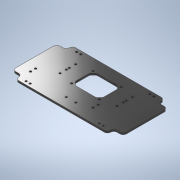
# Autodesk Inventor part: Sole_frame
Saved by Autodesk Inventor 2022.3 (Build 263350000, 350)
## iProperties
Part Number: Sole_frame
Material: GFRP
Document SubType Name: Modeling
Designer: Masato Kubotera
Density: 1.75 g/cm^3
Appearance: 低 光沢 - 黒
Description: GFRP T3
Mass: 67.4649 g
Surface Area: 284.007 cm^2
Volume: 38.5514 cm^3
Author: Masato Kubotera
Revision Number: Rev.2 Specifications for RoboCup 2023: The shape was changed for the installation of load cells.
Autodesk Inventor part; units mm, degrees
ref_plane "YZ Plane" through (0, 0, 0) normal (1, 0, 0) x (0, 1, 0)
ref_plane "XZ Plane" through (0, 0, 0) normal (0, 1, 0) x (-1, 0, 0)
ref_plane "XY Plane" through (0, 0, 0) normal (0, 0, 1) x (1, 0, 0)
sketch "スケッチ1" plane through (0, 0, 0) normal (0, 0, 1) x (1, 0, 0)
  line L0 (-96.735, 64.25) -> (78.265, 64.25)
  line L1 (78.265, 64.25) -> (78.265, -25.75)
  line L2 (78.265, -25.75) -> (-96.735, -25.75)
  line L3 (-96.735, -25.75) -> (-96.735, 64.25)
  line L4 (-96.735, 64.25) -> (78.265, -25.75) construction
  line L5 (78.265, 64.25) -> (-96.735, -25.75) construction
  line L6 (-96.735, 19.25) -> (78.265, 19.25) construction
  line L7 (-96.735, 0) -> (78.265, 0) construction
  line L8 (-80, 4) -> (-80, -4) construction
  circle A0 centre (-80, -4) radius 1.6
  line L9 (0, 64.25) -> (0, -25.75) construction
  line L10 (19, -4) -> (19, 4) construction
  circle A1 centre (19, -4) radius 1.6
  circle A2 centre (-80, 4) radius 1.6
  circle A3 centre (19, 4) radius 1.6
  line L11 (16, 12.5) -> (22, 12.5) construction
  line L12 (22, 12.5) -> (22, -12.5) construction
  line L13 (22, -12.5) -> (16, -12.5) construction
  line L14 (16, -12.5) -> (16, 12.5) construction
  line L15 (16, 12.5) -> (22, -12.5) construction
  line L16 (22, 12.5) -> (16, -12.5) construction
  line L17 (-83, 12.5) -> (-77, 12.5) construction
  line L18 (-77, 12.5) -> (-77, -12.5) construction
  line L19 (-77, -12.5) -> (-83, -12.5) construction
  line L20 (-83, -12.5) -> (-83, 12.5) construction
  line L21 (-83, 12.5) -> (-77, -12.5) construction
  line L22 (-77, 12.5) -> (-83, -12.5) construction
  line L23 (-67, 49.25) -> (6, 49.25) construction
  line L24 (6, 49.25) -> (6, -10.75) construction
  line L25 (6, -10.75) -> (-67, -10.75) construction
  line L26 (-67, -10.75) -> (-67, 49.25) construction
  line L27 (-67, 49.25) -> (6, -10.75) construction
  line L28 (6, 49.25) -> (-67, -10.75) construction
  line L29 (-83, -4.5) -> (-83, 20.5) construction
  line L30 (-83, 20.5) -> (-77, 20.5) construction
  line L31 (-77, 20.5) -> (-77, -4.5) construction
  line L32 (-77, -4.5) -> (-83, -4.5) construction
  circle A4 centre (-80, 12) radius 1.6
  circle A5 centre (-80, 4) radius 1.6
  line L33 (16, 20.5) -> (22, 20.5) construction
  line L34 (16, -4.5) -> (16, 20.5) construction
  line L35 (22, -4.5) -> (16, -4.5) construction
  line L36 (22, 20.5) -> (22, -4.5) construction
  circle A6 centre (19, 4) radius 1.6
  circle A7 centre (19, 12) radius 1.6
  line L37 (-83, 3.5) -> (-83, 28.5) construction
  line L38 (-83, 28.5) -> (-77, 28.5) construction
  line L39 (-77, 28.5) -> (-77, 3.5) construction
  line L40 (-77, 3.5) -> (-83, 3.5) construction
  circle A8 centre (-80, 20) radius 1.6
  circle A9 centre (-80, 12) radius 1.6
  line L41 (16, 28.5) -> (22, 28.5) construction
  line L42 (16, 3.5) -> (16, 28.5) construction
  line L43 (22, 3.5) -> (16, 3.5) construction
  line L44 (22, 28.5) -> (22, 3.5) construction
  circle A10 centre (19, 12) radius 1.6
  circle A11 centre (19, 20) radius 1.6
  circle A12 centre (-80, -12) radius 1.6
  line L45 (-77, -20.5) -> (-83, -20.5) construction
  line L46 (-83, -20.5) -> (-83, 4.5) construction
  line L47 (-77, 4.5) -> (-77, -20.5) construction
  line L48 (16, -20.5) -> (16, 4.5) construction
  circle A13 centre (19, -12) radius 1.6
  line L49 (22, -20.5) -> (16, -20.5) construction
  line L50 (22, 4.5) -> (22, -20.5) construction
  line L51 (45.415, -24.7) -> (77.215, -24.7) construction
  line L52 (77.215, -16.8) -> (45.415, -16.8) construction
  line L53 (45.415, -16.8) -> (45.415, -24.7) construction
  line L54 (45.415, -24.7) -> (77.215, -16.8) construction
  line L55 (77.215, -24.7) -> (45.415, -16.8) construction
  line L56 (77.215, -20.75) -> (45.415, -20.75) construction
  line L57 (61.315, -24.7) -> (61.315, -16.8) construction
  circle A14 centre (45.415, -20.75) radius 1.6
  circle A15 centre (51.765, -20.75) radius 1.6
  line L58 (73.615, -19.1623) -> (73.615, -22.3377) construction
  line L59 (73.615, -22.3377) -> (70.865, -23.9254) construction
  line L60 (70.865, -23.9254) -> (68.115, -22.3377) construction
  line L61 (68.115, -22.3377) -> (68.115, -19.1623) construction
  line L62 (68.115, -19.1623) -> (70.865, -17.5746) construction
  line L63 (70.865, -17.5746) -> (73.615, -19.1623) construction
  line L64 (-9.235, 64.25) -> (-9.235, -25.75) construction
  circle A16 centre (45.415, 59.25) radius 1.6
  circle A17 centre (51.765, 59.25) radius 1.6
  line L65 (73.615, 57.6623) -> (73.615, 60.8377) construction
  line L66 (73.615, 60.8377) -> (70.865, 62.4254) construction
  line L67 (70.865, 62.4254) -> (68.115, 60.8377) construction
  line L68 (68.115, 60.8377) -> (68.115, 57.6623) construction
  line L69 (68.115, 57.6623) -> (70.865, 56.0746) construction
  line L70 (70.865, 56.0746) -> (73.615, 57.6623) construction
  circle A18 centre (-63.885, -20.75) radius 1.6
  circle A19 centre (-70.235, -20.75) radius 1.6
  line L71 (-92.085, -19.1623) -> (-92.085, -22.3377) construction
  line L72 (-92.085, -22.3377) -> (-89.335, -23.9254) construction
  line L73 (-89.335, -23.9254) -> (-86.585, -22.3377) construction
  line L74 (-86.585, -22.3377) -> (-86.585, -19.1623) construction
  line L75 (-86.585, -19.1623) -> (-89.335, -17.5746) construction
  line L76 (-89.335, -17.5746) -> (-92.085, -19.1623) construction
  circle A20 centre (-63.885, 59.25) radius 1.6
  circle A21 centre (-70.235, 59.25) radius 1.6
  line L77 (-86.585, 57.6623) -> (-89.335, 56.0746) construction
  line L78 (-86.585, 60.8377) -> (-86.585, 57.6623) construction
  line L79 (-89.335, 62.4254) -> (-86.585, 60.8377) construction
  line L80 (-92.085, 60.8377) -> (-89.335, 62.4254) construction
  line L81 (-92.085, 57.6623) -> (-92.085, 60.8377) construction
  line L82 (-89.335, 56.0746) -> (-92.085, 57.6623) construction
  line L83 (-34.235, 49.25) -> (15.765, 49.25) construction
  line L84 (15.765, 49.25) -> (15.765, 9.25) construction
  line L85 (15.765, 9.25) -> (-34.235, 9.25) construction
  line L86 (-34.235, 9.25) -> (-34.235, 49.25) construction
  line L87 (-34.235, 49.25) -> (15.765, 9.25) construction
  line L88 (15.765, 49.25) -> (-34.235, 9.25) construction
  line L89 (-31.235, 46.25) -> (12.765, 46.25) construction
  line L90 (12.765, 46.25) -> (12.765, 12.25) construction
  line L91 (12.765, 12.25) -> (-31.235, 12.25) construction
  line L92 (-31.235, 12.25) -> (-31.235, 46.25) construction
  line L93 (-31.235, 46.25) -> (12.765, 12.25) construction
  line L94 (12.765, 46.25) -> (-31.235, 12.25) construction
  circle A22 centre (-31.235, 12.25) radius 1.6
  circle A23 centre (-31.235, 46.25) radius 1.6
  circle A24 centre (12.765, 46.25) radius 1.6
  circle A25 centre (12.765, 12.25) radius 1.6
  line L95 (-62, -21.85) -> (-61.735, -21.85)
  line L96 (77.215, -16.8) -> (77.215, -24.7) construction
  line L97 (63.465, -25.75) -> (63.465, -15.75)
  line L98 (63.465, -15.75) -> (78.265, -15.75)
  line L99 (70.865, -23.9254) -> (70.865, -17.5746) construction
  line L100 (63.465, 64.25) -> (63.465, 54.25)
  line L101 (63.465, 54.25) -> (78.265, 54.25)
  line L102 (-81.935, -25.75) -> (-81.935, -15.75)
  line L103 (-81.935, -15.75) -> (-96.735, -15.75)
  line L104 (-81.935, 54.25) -> (-96.735, 54.25)
  line L105 (-81.935, 64.25) -> (-81.935, 54.25)
  line L106 (-9.235, 49.25) -> (-9.235, 9.25) construction
  circle A26 centre (35.765, 31.5525) radius 1.5
  circle A27 centre (35.765, 41.5525) radius 1.5
  line L107 (35.765, 31.5525) -> (35.765, 41.5525) construction
  line L108 (-34.235, 29.25) -> (15.765, 29.25) construction
  circle A28 centre (35.765, 26.9475) radius 1.5
  circle A29 centre (35.765, 16.9475) radius 1.5
  circle A30 centre (-54.235, 31.5525) radius 1.5
  circle A31 centre (-54.235, 41.5525) radius 1.5
  circle A32 centre (-54.235, 26.9475) radius 1.5
  circle A33 centre (-54.235, 16.9475) radius 1.5
  circle A34 centre (-16.735, -10.75) radius 1.5
  circle A35 centre (-1.735, -10.75) radius 1.5
  line L109 (-1.735, -10.75) -> (-16.735, -10.75) construction
  arc A36 (-27.235, 12.25) -> (-31.235, 16.25) centre (-31.235, 12.25) ccw
  line L110 (-31.235, 16.25) -> (-31.235, 42.25)
  line L111 (-27.235, 12.25) -> (8.765, 12.25)
  arc A37 (12.765, 16.25) -> (8.765, 12.25) centre (12.765, 12.25) ccw
  line L112 (12.765, 16.25) -> (12.765, 42.25)
  arc A38 (-31.235, 42.25) -> (-27.235, 46.25) centre (-31.235, 46.25) ccw
  line L113 (-27.235, 46.25) -> (8.765, 46.25)
  arc A39 (8.765, 46.25) -> (12.765, 42.25) centre (12.765, 46.25) ccw
  point P0 (0, 0)
  point P1 (-9.235, 19.25)
  point P2 (-80, 0)
  point P3 (19, 0)
  point P4 (-30.5, 19.25)
  point P5 (61.315, -20.75)
  point P6 (70.865, -20.75)
  point P7 (-9.235, 29.25)
  point P8 (-9.235, 29.25)
  point P9 (-9.235, 29.25)
  point P10 (35.765, 36.5525)
  point P11 (-9.235, -10.75)
  dimension "d0" = 175
  dimension "d1" = 90
  dimension "d2" = 25.75
  dimension "d3" = 3.2
  dimension "d4" = 8
  dimension "d5" = 8
  dimension "d6" = 3.2
  dimension "d16" = 78.265
  dimension "d17" = 6
  dimension "d18" = 25
  dimension "d19" = 22
  dimension "d20" = 6
  dimension "d21" = 25
  dimension "d22" = 105
  dimension "d23" = 15
  dimension "d24" = 15
  dimension "d25" = 10
  dimension "d26" = 10
  dimension "d57" = 8
  dimension "d64" = 8
  dimension "d69" = 31.8
  dimension "d70" = 7.9
  dimension "d72" = 3.2
  dimension "d75" = 5.5
  dimension "d79" = 50
  dimension "d80" = 40
  dimension "d81" = 44
  dimension "d82" = 34
  dimension "d83" = 3.2
  dimension "d88" = 10
  dimension "d89" = 87.5
  dimension "d102" = 19.1
  dimension "d103" = 5
  dimension "d104" = 1.05
  dimension "d105" = 7.4
  dimension "d106" = 1.05
  dimension "d107" = 3
  dimension "d109" = 20
  dimension "d110" = 10
  dimension "d111" = 7.3025
  dimension "d112" = 42.765
  dimension "d113" = 10
  dimension "d114" = 15
  dimension "d115" = 20
  dimension "d116" = 4
  constraints: 229 end point, 53 symmetric about line, 40 centre point, 32 midpoint, 17 parallel, 13 point on line, 10 horizontal, 10 perpendicular, 8 point on circle, 7 coincident, 7 equal radius, 7 vertical, 4 collinear, 96 other
  measures "d0" distance of L1.end L2.end
  measures "d1" distance of L0.end L1.end
  measures "d2" distance of L2.end L7.start
  measures "d3" diameter of A0
  measures "d4" distance of L8.start L8.end
  measures "d5" distance of L10.start L10.end
  measures "d6" diameter of A1
  measures "d16" distance of L0.end L9.start
  measures "d17" distance of L12.end L13.end
  measures "d18" distance of L11.end L12.end
  measures "d19" horizontal distance of L11.end point (0, 0)
  measures "d20" distance of L18.end L19.end
  measures "d21" distance of L17.end L18.end
  measures "d22" distance of L12.end L19.end
  measures "d23" distance between parallel lines of L23 L0
  measures "d24" distance between parallel lines of L2 L25
  measures "d25" distance between parallel lines of L26 L18
  measures "d26" distance between parallel lines of L14 L24
  measures "d57" distance of L19.end L29.start
  measures "d64" distance of A0.centre A12.centre
  measures "d69" distance of L51.start L51.end
  measures "d70" distance of L52.end L51.start
  measures "d72" diameter of A15
  measures "d75" distance between parallel lines of L60 L63
  measures "d79" distance of L84.end L85.end
  measures "d80" distance of L83.end L84.end
  measures "d81" distance of L90.end L91.end
  measures "d82" distance of L89.end L90.end
  measures "d83" diameter of A22
  measures "d88" distance from line of L6 point (-9.235, 29.25)
  measures "d89" distance from line of point (-9.235, 29.25) L1
  measures "d102" distance of point (70.865, -20.75) A15.centre
  measures "d103" distance from line of L2 L56.end
  measures "d104" distance between parallel lines of L2 L51
  measures "d105" distance from line of L1 point (70.865, -20.75)
  measures "d106" distance between parallel lines of L1 L96
  measures "d107" diameter of A26
  measures "d109" distance between parallel lines of L107 L84
  measures "d110" distance of L107.start L107.end
  measures "d111" vertical distance of point (35.765, 36.552) L108.end
  measures "d112" distance between parallel lines of L39 L86
  measures "d113" distance between parallel lines of L48 L24
  measures "d114" distance of L109.start L109.end
  measures "d115" distance from line of L109.end L85
  measures "d116" radius of A36
extrude "押し出し1" add sketch "スケッチ1" along normal blind 3 contours L0 L100 L101 L1 L98 L97 L2 L102 L103 L3 L104 L105 | A4 | A7 | A8 | A11 | A12 | A13
fillet "フィレット1" radius 5 20 edges at (-81.935, -25.75, 1.5) (-81.935, -15.75, 1.5) (-96.735, -15.75, 1.5) (-96.735, 54.25, 1.5) (-81.935, 54.25, 1.5) (-81.935, 64.25, 1.5) (63.465, 64.25, 1.5) (63.465, 54.25, 1.5) (78.265, 54.25, 1.5) (78.265, -15.75, 1.5) (63.465, -25.75, 1.5) (63.465, -15.75, 1.5) (-27.235, 12.25, 1.5) (-31.235, 16.25, 1.5) (-31.235, 42.25, 1.5) (-27.235, 46.25, 1.5) (8.765, 46.25, 1.5) (12.765, 42.25, 1.5) (12.765, 16.25, 1.5) (8.765, 12.25, 1.5)
equation "\"d3\" = d6"
equation "\"d4\" = d5"
equation "\"d20\" = d17"
equation "\"d21\" = d18"
